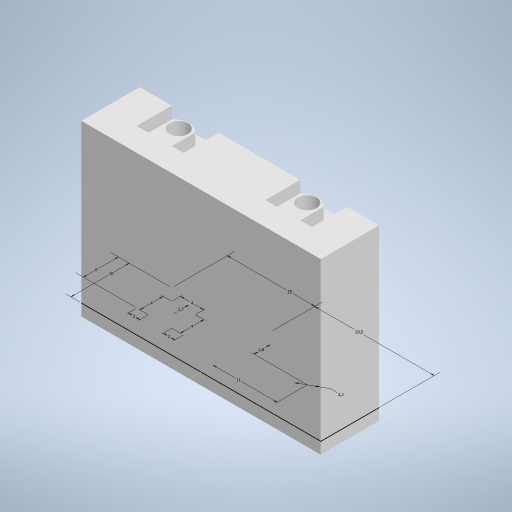
# Autodesk Inventor part: uMule-uchwyt_dx
Saved by Autodesk Inventor 2024.2 (Build 282272000, 272)
## iProperties
Created: 2024-10-21
Part Number: uMule-uchwyt_dx
Material: Ogólny
Document SubType Name: Modeling
Designer: owozn
Density: 1 g/cm^3
Appearance: Domyślna
Author: owozn
Autodesk Inventor part; units mm, degrees
ref_plane "YZ Plane" through (0, 0, 0) normal (1, 0, 0) x (0, 1, 0)
ref_plane "XZ Plane" through (0, 0, 0) normal (0, 1, 0) x (-1, 0, 0)
ref_plane "XY Plane" through (0, 0, 0) normal (0, 0, 1) x (1, 0, 0)
sketch "Szkic1" plane through (0, 0, 0) normal (0, 0, 1) x (1, 0, 0)
  line L0 (-28.7, 0) -> (28.7, 0) construction
  line L1 (0, -17.36) -> (0, 17.36) construction
  line L2 (-20.5, -12.4) -> (20.5, -12.4)
  line L3 (20.5, -12.4) -> (20.5, 12.4)
  line L4 (20.5, 12.4) -> (-20.5, 12.4)
  line L5 (-20.5, 12.4) -> (-20.5, -12.4)
  line L6 (-20.5, -12.4) -> (20.5, 12.4) construction
  line L7 (20.5, -12.4) -> (-20.5, 12.4) construction
  point P0 (0, 0)
  dimension "d0" = 41
  dimension "d1" = 24.8
  constraints: 12 end point, 2 midpoint, 2 parallel, 1 horizontal, 1 perpendicular
  measures "d0" distance of L4.end L3.end
  measures "d1" distance of L3.end L2.end
extrude "Wyciągnięcie proste1" add sketch "Szkic1" along normal blind 10
sketch "Szkic2" plane through (-20.5, -12.4, 0) normal (0, -1, 0) x (1, 0, 0)
  point P0 (20.5, 0)
sketch "Szkic3" plane through (-20.5, -12.4, 0) normal (0, -1, 0) x (1, 0, 0)
  line L0 (-8.2, 0) -> (49.2, 0) construction
  line L1 (20.5, -2) -> (20.5, 12) construction
  line L2 (5.5, 6) -> (5.5, 0)
  line L3 (0, 0) -> (41, 0) projected
  line L4 (5.5, 6) -> (7.5, 6)
  line L5 (7.5, 6) -> (7.5, 2)
  line L6 (7.5, 2) -> (11.5, 2) construction
  line L7 (11.5, 2) -> (11.5, 6)
  line L8 (11.5, 6) -> (13.5, 6)
  line L9 (13.5, 6) -> (13.5, 0)
  line L10 (5.5, 0) -> (13.5, 0)
  line L11 (0, 0) -> (0, 10) projected
  line L12 (0, 0) -> (41, 0)
  line L13 (41, 0) -> (41, 10)
  line L14 (41, 10) -> (0, 10)
  line L15 (0, 10) -> (0, 0)
  arc A0 (7.5, 2) -> (11.5, 2) centre (9.5, 3.8138) ccw
  line L16 (35.5, 6) -> (35.5, 0)
  line L17 (35.5, 6) -> (33.5, 6)
  line L18 (33.5, 6) -> (33.5, 2)
  line L19 (29.5, 2) -> (29.5, 6)
  line L20 (29.5, 6) -> (27.5, 6)
  line L21 (27.5, 6) -> (27.5, 0)
  arc A1 (29.5, 2) -> (33.5, 2) centre (31.5, 3.8138) ccw
  circle A2 centre (31.5, 2.8) radius 1.6
  circle A3 centre (9.5, 2.8) radius 1.6
  point P0 (20.5, 0)
  point P1 (20.5, 0)
  dimension "d4" = 6
  dimension "d5" = 15
  dimension "d6" = 2
  dimension "d7" = 4
  dimension "d8" = 4
  dimension "d9" = 4
  dimension "d10" = 2
  dimension "d11" = 20.5
  dimension "d12" = 10
  dimension "d13" = 2.7
  dimension "d16" = 3.2
  dimension "d17" = 2.8
  dimension "d18" = 11
  constraints: 36 end point, 10 symmetric about line, 6 perpendicular, 4 centre point, 4 point on circle, 2 horizontal, 2 midpoint, 2 parallel, 2 point on line, 1 collinear, 1 vertical, 2 other
  measures "d4" distance of L2.start L2.end
  measures "d5" distance between parallel lines of L1 L2
  measures "d6" distance of L2.start L4.end
  measures "d7" distance of L4.end L5.end
  measures "d8" distance of L5.end L6.end
  measures "d9" distance of L6.end L7.end
  measures "d10" distance of L7.end L8.end
  measures "d11" distance between parallel lines of L13 L1
  measures "d12" distance between parallel lines of L0 L14
  measures "d13" radius of A0
  measures "d16" diameter of A2
  measures "d17" distance from line of L3 A2.centre
  measures "d18" distance from line of L1 A2.centre
extrude "Wyciągnięcie proste2" add sketch "Szkic3" along normal blind 2 and the other way blind 27 contours L2 L3 L11 L14 L13 L16 L17 L18 A1 L19 L20 L21 L9 L8 L7 A0 L5 L4 | A2 | A3
extrude "Wyciągnięcie proste3" cut sketch "Szkic3" along normal through all both and the other way through all contours A2 | A3
